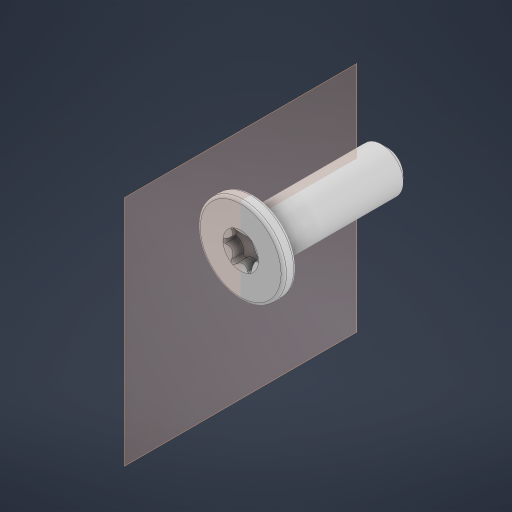
# Autodesk Inventor part: SScrew Star Flat-Head 0.500 SScrew Star Flat-Head 0.500 SScrew Star Flat-Head 0.500 SScrew Star Flat-Head 0.500 SScrew Star Flat-Head 0.500
Saved by Autodesk Inventor 2024.2 (Build 282272000, 272)
## iProperties
Created: 2025-03-21
Part Number: SScrew Star Flat-Head 0.500 SScrew Star Flat-Head 0.500 SScrew Star Flat-Head 0.500 SScrew Star Flat-Head 0.500 SScrew Star Flat-Head 0.500
Material: Generic
Document SubType Name: Modeling
Designer: AdityaSingh
Density: 1 g/cm^3
Appearance: Default
Author: AdityaSingh
Autodesk Inventor part; units mm, degrees
ref_plane "YZ Plane" through (0, 0, 0) normal (1, 0, 0) x (0, 1, 0)
ref_plane "XZ Plane" through (0, 0, 0) normal (0, 1, 0) x (-1, 0, 0)
ref_plane "XY Plane" through (0, 0, 0) normal (0, 0, 1) x (1, 0, 0)
sketch "Sketch1" plane through (0, 0, 0) normal (0, 0, 1) x (1, 0, 0)
  circle A0 centre (0, 0) radius 4.0767
  dimension "d0" = 8.1534
  constraints: 1 centre point, 1 coincident
  measures "d0" diameter of A0
extrude "Extrusion1" add sketch "Sketch1" along normal blind 1.1938
fillet "Fillet2" radius 0.254 2 edges at (-4.0767, 0, 1.1938) (-4.0767, 0, 0)
sketch "Sketch3" plane through (0, 0, 1.1938) normal (0, 0, 1) x (1, 0, 0)
  circle A0 centre (0, 0) radius 1.6764 construction
  line L0 (0, 0) -> (1.6764, 0) construction
  line L1 (0, 0) -> (-1.6764, 0) construction
  line L2 (0, 0) -> (0.8382, -1.4518) construction
  line L3 (0, 0) -> (0.8382, 1.4518) construction
  line L4 (0, 0) -> (-0.8382, 1.4518) construction
  line L5 (0, 0) -> (-0.8382, -1.4518) construction
  circle A1 centre (0, 0) radius 1.4605 construction
  circle A2 centre (1.4605, 0) radius 0.2159 construction
  circle A3 centre (0.7303, -1.2648) radius 0.2159 construction
  circle A4 centre (-0.7303, -1.2648) radius 0.2159 construction
  circle A5 centre (-1.4605, 0) radius 0.2159 construction
  circle A6 centre (-0.7303, 1.2648) radius 0.2159 construction
  circle A7 centre (0.7302, 1.2648) radius 0.2159 construction
  circle A8 centre (0, 0) radius 2.0701 construction
  line L6 (1.7928, -1.0351) -> (0, 0) construction
  circle A9 centre (0, 0) radius 1.1989 construction
  circle A10 centre (1.7928, -1.0351) radius 0.8712 construction
  line L7 (0, 0) -> (1.7928, 1.0351) construction
  circle A11 centre (1.7928, 1.0351) radius 0.8712 construction
  arc A12 (1.5265, -0.2056) -> (0.9413, -1.2192) centre (1.7928, -1.0351) ccw
  arc A13 (1.5265, -0.2056) -> (1.5265, 0.2056) centre (1.4605, 0) ccw
  arc A14 (0.9413, 1.2192) -> (1.5265, 0.2056) centre (1.7928, 1.0351) ccw
  line L8 (0, 0) -> (0, 2.0701) construction
  line L9 (0, 0) -> (0, -2.0701) construction
  line L10 (0, 0) -> (-1.7928, -1.0351) construction
  line L11 (0, 0) -> (-1.7928, 1.0351) construction
  circle A15 centre (0, 2.0701) radius 0.8712 construction
  circle A16 centre (-1.7928, 1.0351) radius 0.8712 construction
  circle A17 centre (-1.7928, -1.0351) radius 0.8712 construction
  circle A18 centre (0, -2.0701) radius 0.8712 construction
  arc A19 (-0.5852, 1.4248) -> (0.5852, 1.4248) centre (0, 2.0701) ccw
  arc A20 (0.9413, 1.2192) -> (0.5852, 1.4248) centre (0.7303, 1.2648) ccw
  arc A21 (-0.5852, 1.4248) -> (-0.9413, 1.2192) centre (-0.7303, 1.2648) ccw
  arc A22 (-1.5265, 0.2056) -> (-0.9413, 1.2192) centre (-1.7928, 1.0351) ccw
  arc A23 (-1.5265, 0.2056) -> (-1.5265, -0.2056) centre (-1.4605, 0) ccw
  arc A24 (-0.9413, -1.2192) -> (-1.5265, -0.2056) centre (-1.7928, -1.0351) ccw
  arc A25 (-0.9413, -1.2192) -> (-0.5852, -1.4248) centre (-0.7303, -1.2648) ccw
  arc A26 (0.5852, -1.4248) -> (-0.5852, -1.4248) centre (0, -2.0701) ccw
  arc A27 (0.5852, -1.4248) -> (0.9413, -1.2192) centre (0.7303, -1.2648) ccw
  dimension "d6" = 3.3528
  dimension "d7" = 60
  dimension "d8" = 60
  dimension "d9" = 60
  dimension "d10" = 2.921
  dimension "d11" = 0.4318
  dimension "d12" = 0.4318
  dimension "d13" = 0.4318
  dimension "d14" = 0.4318
  dimension "d15" = 4.1402
  dimension "d16" = 30
  dimension "d17" = 2.3979
  dimension "d18" = 30
  dimension "d19" = 30
  dimension "d20" = 30
  constraints: 70 point on circle, 28 centre point, 24 end point, 10 coincident, 9 point on line, 2 tangent, 1 concentric, 1 horizontal, 1 vertical
  measures "d6" diameter of A0
  measures "d7" angle of L1 L5
  measures "d8" angle of L0 L2
  measures "d9" angle of L1 L4
  measures "d10" diameter of A1
  measures "d11" diameter of A2
  measures "d12" diameter of A3
  measures "d13" diameter of A4
  measures "d14" diameter of A5
  measures "d15" diameter of A8
  measures "d16" angle of L0 L6
  measures "d17" diameter of A9
  measures "d18" angle of L3 L7
  measures "d19" angle of L5 L10
  measures "d20" angle of L4 L11
extrude "Extrusion2" cut sketch "Sketch3" against normal blind 1.4963
sketch "Sketch4" plane through (0, 0, 1.1938) normal (0, 0, 1) x (1, 0, 0)
  circle A0 centre (0, 0) radius 1.6764 construction
  circle A1 centre (0, 0) radius 1.6764
  line L0 (0, -1.6764) -> (0, 1.6764)
  line L1 (-1.6764, -1.6764) -> (1.353, -1.6764)
  line L2 (1.353, -1.6764) -> (1.353, 1.6764)
  line L3 (1.353, 1.6764) -> (-1.6764, 1.6764)
  line L4 (-1.6764, 1.6764) -> (-1.6764, -1.6764)
  constraints: 10 end point, 3 tangent, 2 parallel, 2 point on circle, 1 centre point, 1 coincident, 1 concentric, 1 horizontal, 1 perpendicular, 1 vertical
sketch "Sketch6" plane through (0, 0, 0) normal (0, 0, -1) x (-1, 0, 0)
  circle A0 centre (0, 0) radius 2.0828
  circle A1 centre (0, 0) radius 1.4859
  dimension "d23" = 4.1656
  dimension "d24" = 2.9718
  constraints: 2 centre point, 2 coincident
  measures "d23" diameter of A0
  measures "d24" diameter of A1
extrude "Extrusion4" add sketch "Sketch6" along normal blind 12.7 contours A0 | A1
chamfer "Chamfer1" distance 0.5969 angle 45 1 edges at (2.0828, 0, -12.7)
sketch "Sketch7" plane through (0, 0, 1.1938) normal (0, 0, 1) x (1, 0, 0)
  line L0 (-0.2259, -1.1613) -> (0, -1.1613)
  line L1 (0, -1.1613) -> (0, 1.1378)
  line L2 (0, 1.1378) -> (-0.2259, 1.1378)
  line L3 (-0.2259, 1.1378) -> (-0.2259, -1.1613)
  point P0 (0, 0)
  dimension "d33" = 0.226
  dimension "d34" = 2.2991
  constraints: 8 end point, 2 parallel, 1 horizontal, 1 perpendicular, 1 point on line
  measures "d33" distance of L1.end L2.end
  measures "d34" distance of L2.end L0.start
ref_plane "Work Plane1" through (0, -1.1613, 1.1938) normal (1, 0, 0) x (0, 0, -1)
sketch "Sketch9" plane through (0, -1.1613, 1.1938) normal (1, 0, 0) x (0, 0, -1)
  line L0 (0, 2.8377) -> (0, -0.5151) construction
  line L1 (0, 1.1613) -> (0, 2.8377)
  line L2 (0, 1.1613) -> (0.889, 1.1613)
  line L3 (0.889, 1.1613) -> (0, 2.8377)
  point P0 (1.1938, 1.1613)
  dimension "d39" = 0.889
  constraints: 6 end point, 1 collinear, 1 horizontal
  measures "d39" distance of L1.start L2.end
revolve "Revolution2" cut sketch "Sketch9" angle 360 about axis through (0, 0, 1.1938) along (0, 0, -1)
body "Solid1"
